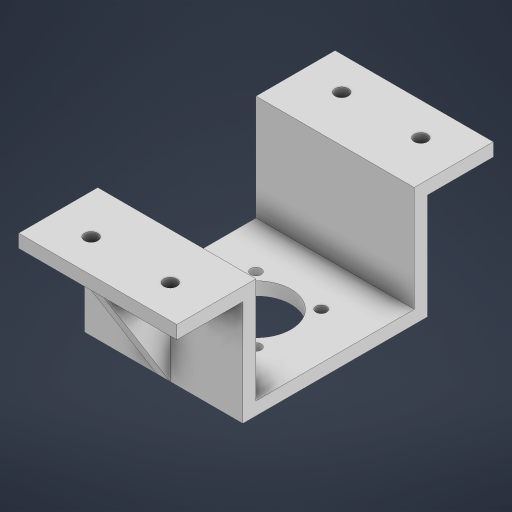
# Autodesk Inventor part: Base_Motor_Mount
Saved by Autodesk Inventor 2023 (Build 270158000, 158)
## iProperties
Created: 2023-09-15
Part Number: Base_Motor_Mount
Material: Generic
Document SubType Name: Modeling
Designer: Abhinav
Density: 1 g/cm^3
Appearance: Default
Author: Abhinav
Autodesk Inventor part; units mm, degrees
ref_plane "YZ Plane" through (0, 0, 0) normal (1, 0, 0) x (0, 1, 0)
ref_plane "XZ Plane" through (0, 0, 0) normal (0, 1, 0) x (-1, 0, 0)
sketch "Sketch1" plane through (0, 0, 0) normal (0, 1, 0) x (-1, 0, 0)
  circle A0 centre (0, 0) radius 13.25
  line L0 (0, 0) -> (12.3744, 12.3744) construction
  line L1 (0, 0) -> (17.5, 0) construction
  line L2 (0, 0) -> (-12.3744, -12.3744) construction
  line L3 (0, 0) -> (17.5, 0) construction
  circle A1 centre (-12.3744, -12.3744) radius 2
  circle A2 centre (12.3744, 12.3744) radius 2
  circle A3 centre (12.3744, -12.3744) radius 2
  circle A4 centre (-12.3744, 12.3744) radius 2
  circle A5 centre (0, 0) radius 17.5 construction
  line L4 (30, 30) -> (-30, 30)
  line L5 (-30, 30) -> (-30, -30)
  line L6 (-30, -30) -> (30, -30)
  line L7 (30, -30) -> (30, 30)
  line L8 (30, 30) -> (-30, -30) construction
  line L9 (-30, 30) -> (30, -30) construction
  line L10 (30, -30) -> (-30, -30)
  line L11 (-30, -30) -> (-30, -35)
  line L12 (-30, -35) -> (30, -35)
  line L13 (30, -35) -> (30, -30)
  line L14 (30, 30) -> (-30, 30)
  line L15 (-30, 30) -> (-30, 35)
  line L16 (-30, 35) -> (30, 35)
  line L17 (30, 35) -> (30, 30)
  dimension "d0" = 26.5
  dimension "d1" = 17.5
  dimension "d2" = 45
  dimension "d3" = 17.5
  dimension "d4" = 135
  dimension "d5" = 4
  dimension "d6" = 4
  dimension "d7" = 60
  dimension "d9" = 5
  dimension "d10" = 5
  constraints: 36 end point, 6 parallel, 5 centre point, 5 horizontal, 4 coincident, 3 equal length, 3 perpendicular, 2 midpoint, 2 symmetric about line, 1 point on line, 5 other
  measures "d0" diameter of A0
  measures "d1" distance of L0.start L0.end
  measures "d2" angle of L1 L0
  measures "d3" distance of L0.start L2.end
  measures "d4" angle of L2 L3
  measures "d5" diameter of A1
  measures "d6" diameter of A2
  measures "d7" distance of L6.end L5.end
  measures "d9" distance of L11.end L10.end
  measures "d10" distance of L14.end L15.end
extrude "Extrusion1" add sketch "Sketch1" against normal blind 5
extrude "Extrusion2" add sketch "Sketch1" along normal blind 35 contours L4 L15 L16 L17 | L13 L12 L11 L6
sketch "Sketch4" plane through (-30, 35, 30) normal (0, 1, 0) x (1, 0, 0)
  line L0 (0, 60) -> (0, 0) construction
  line L1 (0, -30) -> (60, -30) construction
  line L2 (30, -17.5) -> (45, -17.5) construction
  line L3 (60, -5) -> (60, -30) construction
  line L4 (30, -17.5) -> (15, -17.5) construction
  circle A0 centre (45, -17.5) radius 2.5
  circle A1 centre (15, -17.5) radius 2.5
  line L5 (60, 0) -> (0, 0) projected
  line L6 (0, 0) -> (0, -30) projected
  line L7 (60, -30) -> (0, -30) projected
  line L8 (60, 0) -> (60, -30) projected
  line L9 (0, 60) -> (60, 60)
  line L10 (60, 60) -> (60, 90)
  line L11 (60, 90) -> (0, 90)
  line L12 (0, 90) -> (0, 60)
  line L13 (60, 0) -> (0, 0) projected
  line L14 (0, 0) -> (60, 0)
  line L15 (60, -5) -> (0, -5) projected
  line L16 (60, -30) -> (0, -30)
  line L17 (0, -30) -> (0, -5)
  line L18 (0, -5) -> (60, -5)
  line L19 (60, -5) -> (60, -30)
  line L20 (60, -30) -> (0, -5) construction
  line L21 (30, -17.5) -> (30, -30) construction
  line L22 (30, 77.5) -> (45, 77.5) construction
  line L23 (30, 77.5) -> (15, 77.5) construction
  circle A2 centre (45, 77.5) radius 2.5
  circle A3 centre (15, 77.5) radius 2.5
  line L24 (60, 65) -> (0, 65)
  line L25 (0, 65) -> (0, 90)
  line L26 (0, 90) -> (60, 90)
  line L27 (60, 90) -> (60, 65)
  line L28 (60, 65) -> (0, 90) construction
  line L29 (30, 77.5) -> (30, 65) construction
  point P0 (30, 30)
  dimension "d19" = 15
  dimension "d20" = 5
  dimension "d28" = 15
  dimension "d29" = 5
  constraints: 42 end point, 7 equal length, 5 horizontal, 4 centre point, 4 coincident, 4 midpoint, 4 perpendicular, 2 collinear, 2 equal radius
  measures "d19" distance of L2.start L2.end
  measures "d20" diameter of A0
  measures "d28" distance of L23.start L22.end
  measures "d29" diameter of A2
extrude "Extrusion4" add sketch "Sketch4" along normal blind 5
ref_plane "Work Plane3" through (0, -5, 35) normal (1, 0, 0) x (0, 0, -1)
sketch "Sketch5" plane through (0, -5, 35) normal (1, 0, 0) x (0, 0, -1)
  line L0 (0, 40) -> (0, 0) projected
  line L1 (0, 0) -> (0, 40)
  line L2 (0, 40) -> (-25, 40)
  line L3 (-25, 45) -> (5, 45) projected
  line L4 (-25, 40) -> (0, 0)
  line L5 (0, 0) -> (70, 0) projected
  line L6 (70, 0) -> (70, 40) projected
  line L7 (70, 0) -> (70, 40)
  line L8 (95, 40) -> (70, 40) projected
  line L9 (70, 40) -> (95, 40)
  line L10 (95, 40) -> (70, 0)
  point P0 (35, 5)
  constraints: 12 end point, 1 collinear, 1 parallel, 1 perpendicular, 1 vertical
extrude "Extrusion5" add sketch "Sketch5" along normal mid plane 5
body "Solid1"
